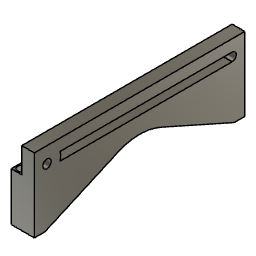
guia v5 brazo (Autodesk Fusion 360 design; units mm, degrees)
Autodesk Fusion 360 part; units mm, degrees
sketch "Sketch1" plane through (0, 0, 0) normal (1, 0, 0) x (0, 1, 0)
  line L0 (0, 0) -> (100, 0)
  line L1 (100, 0) -> (100, 15)
  line L2 (100, 15) -> (0, 15)
  line L3 (0, 15) -> (0, 0)
  dimension "d1" = 100
  dimension "d2" = 15
  constraint horizontal L0
  constraint vertical L1
  constraint horizontal L2
  constraint vertical L3
  constraint coincident L0.start L3.end
  measures "d1" distance of L0.start L0.end
  measures "d2" distance of L0.start L2.end
extrude "Extrude1" add sketch "Sketch1" along normal blind 6
sketch "Sketch2" plane through (6, 0, 0) normal (1, 0, 0) x (0, 1, 0)
  line L0 (0, 15) -> (0, 0)
  line L1 (0, 0) -> (100, 0)
  line L2 (100, 0) -> (100, 15)
  line L3 (100, 15) -> (0, 15)
  circle A0 centre (6, 7.5) radius 4
  circle A1 centre (94, 7.5) radius 4
  line L4 (6, 11.5) -> (94, 11.5)
  line L5 (94, 3.5) -> (6, 3.5)
  circle A2 centre (6, 7.5) radius 6.5013
  dimension "d5" = 8
  dimension "d6" = 6
  dimension "d7" = 8
  dimension "d8" = 6
  constraint coincident A0 L4.start
  constraint coincident A1 L4.end
  constraint tangent A1 L4
  constraint perpendicular L2 L4
  constraint coincident A1 L5.start
  constraint coincident A0 L5.end
  constraint tangent A0 L5
  constraint parallel L1 L5
  constraint concentric A0 A2
  measures "d5" diameter of A0
  measures "d6" distance of L0 A0.centre
  measures "d7" diameter of A1
  measures "d8" distance of L2 A1.centre
extrude "Extrude2" cut sketch "Sketch2" against normal blind 20 contours A1 L4 L5 A2 | A0 | A1
sketch "Sketch3" plane through (0, 0, 0) normal (-1, 0, 0) x (0, -1, 0)
  line L0 (-11.1251, 3.5) -> (-94, 3.5)
  arc A0 (-94, 11.5) -> (-94, 3.5) centre (-94, 7.5) ccw
  line L1 (-94, 11.5) -> (-11.1251, 11.5)
  line L2 (0, 0) -> (0, 15)
  line L3 (0, 15) -> (-100, 15)
  line L4 (-100, 15) -> (-100, 0)
  line L5 (-100, 0) -> (0, 0)
  circle A1 centre (-6, 7.5) radius 4
  arc A2 (-11.1251, 11.5) -> (-11.1251, 3.5) centre (-6, 7.5) ccw
sketch "Sketch4" plane through (0, 50, 7.5) normal (-1, 0, 0) x (0, -1, 0)
sketch "Sketch5" plane through (0, 0, 0) normal (0, 0, -1) x (1, 0, 0)
  line L0 (0, 0) -> (0, -100)
  line L1 (0, -100) -> (6, -100)
  line L2 (6, -100) -> (6, 0)
  line L3 (6, 0) -> (0, 0)
  line L4 (0, -100) -> (-5, -100)
  line L5 (-5, -100) -> (-5, -95)
  line L6 (-5, -95) -> (0, -95)
  line L7 (0, -95) -> (0, -100)
  line L8 (0, 0) -> (-5, 0)
  line L9 (-5, 0) -> (-5, -5)
  line L10 (-5, -5) -> (0, -5)
  line L11 (0, -5) -> (0, 0)
  dimension "d11" = 5
  dimension "d12" = 5
  dimension "d13" = 5
  dimension "d14" = 5
  constraint horizontal L4
  constraint vertical L5
  constraint horizontal L6
  constraint vertical L7
  constraint coincident L0.end L1.start
  constraint horizontal L8
  constraint vertical L9
  constraint horizontal L10
  constraint vertical L11
  constraint coincident L0.start L3.end
  measures "d11" distance of L0.end L4.end
  measures "d12" distance of L0.end L6.end
  measures "d13" distance of L0.start L8.end
  measures "d14" distance of L0.start L10.end
extrude "Extrude3" add sketch "Sketch5" against normal blind 3 contours L0 L8 L9 L10 L11 | L0 L4 L5 L6 L7
sketch "Sketch6" plane through (0, 0, 3) normal (0, 0, 1) x (-1, 0, 0)
  line L0 (5, -95) -> (0, -95)
  line L1 (0, -95) -> (0, -100)
  line L2 (0, -100) -> (5, -100)
  line L3 (5, -100) -> (5, -95)
  circle A0 centre (2.5, -97.5) radius 2
  dimension "d17" = 4
  measures "d17" diameter of A0
extrude "Extrude4" cut sketch "Sketch6" against normal blind 6 contours A0
sketch "Sketch7" plane through (0, 0, 0) normal (-1, 0, 0) x (0, -1, 0)
sketch "Sketch8" plane through (0, 0, 3) normal (0, 0, 1) x (-1, 0, 0)
  line L0 (0, 0) -> (0, -5)
  line L1 (0, -5) -> (5, -5)
  line L2 (5, -5) -> (5, 0)
  line L3 (5, 0) -> (0, 0)
  circle A0 centre (2.5, -2.5) radius 2
  dimension "d20" = 4
  measures "d20" diameter of A0
extrude "Extrude5" cut sketch "Sketch8" against normal blind 9 contours A0
sketch "Sketch9" plane through (0, 50.3094, 7.5) normal (-1, 0, 0) x (0, -1, 0)
extrude "Extrude6" add 1 faces at (4, 65, 0) along direction (0, 0, -1) blind 20
sketch "Sketch10" plane through (0, 0, 0) normal (-1, 0, 0) x (0, -1, 0)
  line L0 (-5, 3) -> (0, 3)
  line L1 (0, 3) -> (0, 15)
  line L2 (0, 15) -> (-100, 15)
  line L3 (-100, 15) -> (-100, 3)
  line L4 (-100, 3) -> (-95, 3)
  line L5 (-95, 3) -> (-95, -20)
  line L6 (-95, -20) -> (-5, -20)
  line L7 (-5, -20) -> (-5, 3)
  circle A0 centre (-6, 7.5) radius 4
  line L8 (-94, 11.5) -> (-11.1251, 11.5)
  arc A1 (-11.1251, 11.5) -> (-11.1251, 3.5) centre (-6, 7.5) ccw
  line L9 (-11.1251, 3.5) -> (-94, 3.5)
  arc A2 (-94, 11.5) -> (-94, 3.5) centre (-94, 7.5) ccw
  line L10 (-95, -20) -> (-50, 0)
  line L11 (-50, 0) -> (-5, -20)
  constraint coincident L5.end L6.start
  constraint coincident L6.end L7.start
extrude "Extrude7" cut sketch "Sketch10" against normal blind 25 contours L6 L10 L11
fillet "Fillet1" radius 25 1 edges at (3, 50, 0)
sketch "Sketch11" plane through (6, 0, 0) normal (1, 0, 0) x (0, 1, 0)
  line L0 (5, -20) -> (39.8465, -4.5126)
  arc A0 (60.1535, -4.5126) -> (39.8465, -4.5126) centre (50, -27.3579) ccw
  line L1 (60.1535, -4.5126) -> (95, -20)
  line L2 (95, -20) -> (100, -20)
  line L3 (100, -20) -> (100, 15)
  line L4 (100, 15) -> (0, 15)
  line L5 (0, 15) -> (0, -20)
  line L6 (0, -20) -> (5, -20)
  line L7 (11.1251, 11.5) -> (94, 11.5)
  arc A1 (94, 3.5) -> (94, 11.5) centre (94, 7.5) ccw
  line L8 (94, 3.5) -> (11.1251, 3.5)
  arc A2 (11.1251, 3.5) -> (11.1251, 11.5) centre (6, 7.5) ccw
  circle A3 centre (6, 7.5) radius 4
  circle A4 centre (6, 7.5) radius 2
  circle A5 centre (94, 7.5) radius 2
  line L9 (94, 9.5) -> (12.186, 9.5)
  line L10 (94, 5.5) -> (12.186, 5.5)
  dimension "d29" = 4
  dimension "d30" = 4
  constraint concentric A2 A4
  constraint concentric A1 A5
  constraint coincident A5 L9.start
  constraint coincident A2 L9.end
  constraint tangent A5 L9
  constraint parallel L7 L9
  constraint coincident A5 L10.start
  constraint coincident A2 L10.end
  constraint tangent A5 L10
  constraint parallel L7 L10
  measures "d29" diameter of A4
  measures "d30" diameter of A5
extrude "Extrude8" add sketch "Sketch11" against normal blind 6 contours L7 A1 L8 A2 A5 L9 L10 | A3
